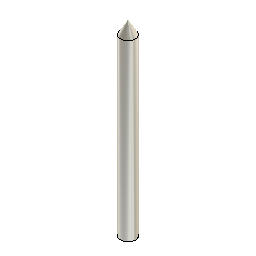
EOAT+Reference+Setup+Tool (Autodesk Fusion 360 design; units mm, degrees)
Autodesk Fusion 360 part; units mm, degrees
sketch "Sketch1" plane through (0, 0, 0) normal (0, 1, 0) x (1, 0, 0)
  line L0 (0, 0) -> (6, 0)
  line L1 (6, 0) -> (6, -150)
  line L2 (6, -150) -> (0, -150)
  line L3 (0, -150) -> (0, 0)
  line L4 (0, -150) -> (6, -139.6077)
  dimension "d1" = 12
  dimension "d2" = 150
  dimension "d3" = 30
  constraint horizontal L0
  constraint vertical L1
  constraint horizontal L2
  constraint vertical L3
  constraint coincident L0.start L3.end
  constraint coincident L1 L4.end
  measures "d2" distance of L0.end L1.end
  measures "d3" angle of L3 L4
revolve "Revolve1" add sketch "Sketch1" angle 360 about axis through (0, 0, 150) along (0, 0, -1) contours L0 L1 L3 L4
hole "Hole1" at (0, 0, 0) direction (0, 0, 1) diameter 5.035 depth 15 tip angle 118
thread "Thread1" "ISO Metric profile 6.0 M6x1 6H"
chamfer "Chamfer1" distance 0.5 angle 45 1 edges at (-5.594, -2.1697, 0)
